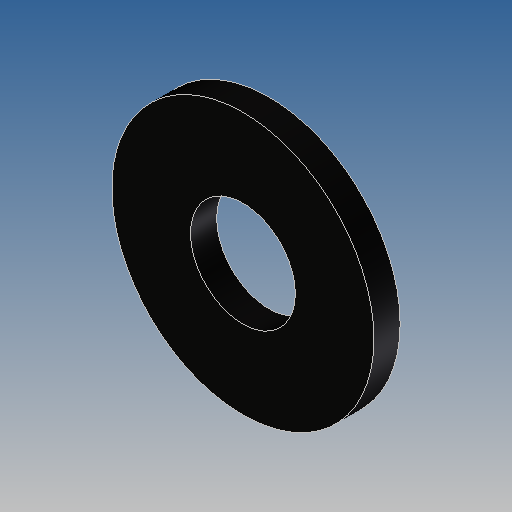
# Autodesk Inventor part: Small Washer
Saved by Autodesk Inventor 2018 (Build 220112000, 112)
## iProperties
Created: 2018-03-28
Part Number: Small Washer
Material: Stainless Steel
Document SubType Name: Modeling
Designer: Cole
Density: 8 g/cm^3
Appearance: Stainless - Brushed
Mass: 4.42823 g
Surface Area: 7.26416 cm^2
Volume: 0.553529 cm^3
Author: Cole
Autodesk Inventor part; units mm, degrees
ref_plane "YZ Plane" through (0, 0, 0) normal (1, 0, 0) x (0, 1, 0)
ref_plane "XZ Plane" through (0, 0, 0) normal (0, 1, 0) x (-1, 0, 0)
ref_plane "XY Plane" through (0, 0, 0) normal (0, 0, 1) x (1, 0, 0)
sketch "Sketch1" plane through (0, 0, 0) normal (0, 0, 1) x (1, 0, 0)
  circle A0 centre (0, 0) radius 10.16
  circle A1 centre (0, 0) radius 4.064
  dimension "d0" = 20.32
  dimension "d1" = 8.128
  constraints: 2 centre point, 2 coincident
  measures "d0" diameter of A0
  measures "d1" diameter of A1
extrude "Extrusion1" add sketch "Sketch1" along normal blind 2.032
body "Solid1"
